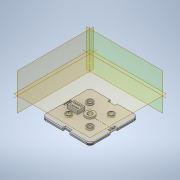
# Autodesk Inventor part: brick_bottom_standard
Saved by Autodesk Inventor 2021 (Build 250183000, 183)
## iProperties
Created: 2025-08-13
Part Number: brick_bottom_standard
Material: Generisch
Document SubType Name: Modeling
Designer: pasca
Density: 1 g/cm^3
Appearance: Vorgabe
Author: pasca
Autodesk Inventor part; units mm, degrees
sketch "Skizze1" plane through (27.583261, -56.113234, -10.899999) normal (0, 0, 1) x (1, 0, 0)
  line L0 (20.486741, 28.426785) -> (20.486741, 31.173234)
  line L1 (28.486738, 28.426785) -> (20.486741, 28.426785)
  line L2 (28.486738, 31.173234) -> (28.486738, 28.426785)
  circle A0 centre (48.116381, 27.672954) radius 3.500451
  line L3 (48.870292, 0.100002) -> (48.870292, 7.94323)
  line L4 (48.973479, 8.043232) -> (51.613555, 8.043232)
  line L5 (51.613555, 0) -> (48.973479, 0)
  circle A1 centre (48.116472, -19.586583) radius 3.50032
  line L6 (20.529933, -20.340319) -> (28.529944, -20.340319)
  line L7 (28.529944, -20.340319) -> (28.529944, -23.086762)
  line L8 (20.529933, -23.086762) -> (20.529933, -20.340319)
  circle A2 centre (0.857019, -19.586408) radius 3.500451
  line L9 (0.103188, 7.94323) -> (0.103188, 0.100002)
  line L10 (-2.640073, 8.043232) -> (0, 8.043232)
  line L11 (0, 0) -> (-2.640073, 0)
  circle A3 centre (0.856903, 27.67302) radius 3.50027
  circle A4 centre (6.691673, 3.973123) radius 1.000129
  circle A5 centre (9.236925, 3.973204) radius 1.000185
  circle A6 centre (11.781701, 3.973221) radius 0.999961
  circle A7 centre (14.326498, 3.973153) radius 0.999748
  circle A8 centre (14.3269, 0.233503) radius 0.99969
  circle A9 centre (11.78165, 0.233145) radius 1.000125
  circle A10 centre (9.236749, 0.233322) radius 0.999912
  circle A11 centre (6.691637, 0.232928) radius 1.000319
  line L12 (-2.640073, 8.043232) -> (0.103188, 8.043232)
  line L13 (0.103188, 8.043232) -> (0.103188, 0)
  line L14 (0.103188, 0) -> (-2.640073, 0)
  line L15 (20.486741, 31.173234) -> (20.486741, 28.426785)
  line L16 (28.486738, 28.426785) -> (28.486738, 31.173234)
  line L17 (48.116736, 31.173234) -> (28.486738, 31.173234)
  line L18 (0.85674, -23.086762) -> (20.529933, -23.086762)
  line L19 (-2.643261, 0.100002) -> (-2.643261, -19.586763)
  line L20 (51.616735, -19.586763) -> (51.616735, 0.100002)
  line L21 (-2.643261, 27.673233) -> (-2.643261, 7.94323)
  line L22 (20.486741, 31.173234) -> (0.85674, 31.173234)
  line L23 (51.616735, 7.94323) -> (51.616735, 27.673233)
  line L24 (28.529944, -23.086762) -> (48.116736, -23.086762)
  line L25 (-2.643261, -23.086762) -> (51.616735, -23.086762)
  line L26 (51.616735, -23.086762) -> (51.616735, 31.173234)
  line L27 (51.616735, 31.173234) -> (-2.643261, 31.173234)
  line L28 (-2.643261, 31.173234) -> (-2.643261, -23.086762)
  line L29 (51.613555, 8.043232) -> (48.870292, 8.043232)
  line L30 (48.870292, 8.043232) -> (48.870292, 0)
  line L31 (48.870292, 0) -> (51.613555, 0)
  line L32 (48.870292, 0) -> (51.613555, 0)
  line L33 (48.870292, 0) -> (48.870292, 8.043232)
  line L34 (51.613555, 8.043232) -> (48.870292, 8.043232)
  line L35 (48.870292, 8.043232) -> (48.870292, 0)
  line L36 (48.870292, 0) -> (51.613555, 0)
  line L37 (51.613555, 0) -> (51.613555, 8.043232)
  line L38 (0.103188, 0) -> (-2.640073, 0)
  line L39 (-2.640073, 8.043232) -> (0.103188, 8.043232)
  line L40 (0.103188, 0) -> (-2.640073, 0)
  line L41 (-2.640073, 0) -> (-2.640073, 8.043232)
  line L42 (-2.640073, 8.043232) -> (0.103188, 8.043232)
  line L43 (0.103188, 8.043232) -> (0.103188, 0)
  point P0 (-27.583261, 56.113234)
  point P1 (0.837182, 31.173234)
  point P2 (-2.643261, 27.700217)
  point P3 (-2.643261, -19.621008)
  point P4 (0.830931, -23.086762)
  point P5 (48.147826, -23.086762)
  point P6 (51.616735, -19.606381)
  point P7 (51.616735, 27.699042)
  point P8 (48.150981, 31.173234)
  constraints: 48 end point, 6 perpendicular, 5 collinear, 4 horizontal, 4 parallel, 3 point on line, 1 vertical
sketch "Skizze1 outline for Extrusion2" plane through (27.583261, -56.113234, -10.899999) normal (0, 0, 1) x (1, 0, 0)
  line L0 (28.486738, 28.426785) -> (20.486741, 28.426785)
  line L1 (28.486738, 31.173234) -> (28.486738, 28.426785)
  line L2 (20.486741, 28.426785) -> (20.486741, 31.173234)
  line L3 (48.116736, 31.173234) -> (28.486738, 31.173234)
  line L4 (20.486741, 31.173234) -> (0.85674, 31.173234)
  line L5 (48.150981, 31.173234) -> (48.116736, 31.173234)
  line L6 (0.85674, 31.173234) -> (0.837182, 31.173234)
  arc A0 (51.616735, 27.699042) -> (48.150981, 31.173234) centre (48.116381, 27.672954) ccw
  arc A1 (0.837182, 31.173234) -> (-2.643261, 27.700217) centre (0.856903, 27.67302) ccw
  line L7 (51.616735, 27.673233) -> (51.616735, 27.699042)
  line L8 (-2.643261, 27.700217) -> (-2.643261, 27.673233)
  line L9 (51.616735, 7.94323) -> (51.616735, 27.673233)
  line L10 (-2.643261, 27.673233) -> (-2.643261, 7.94323)
  line L11 (51.616735, 0.100002) -> (51.616735, 7.94323)
  line L12 (-2.643261, 7.94323) -> (-2.643261, 0.100002)
  line L13 (51.616735, -19.586763) -> (51.616735, 0.100002)
  line L14 (-2.643261, 0.100002) -> (-2.643261, -19.586763)
  line L15 (51.616735, -19.606381) -> (51.616735, -19.586763)
  line L16 (-2.643261, -19.586763) -> (-2.643261, -19.621008)
  arc A2 (48.147826, -23.086762) -> (51.616735, -19.606381) centre (48.116472, -19.586583) ccw
  arc A3 (-2.643261, -19.621008) -> (0.830931, -23.086762) centre (0.857019, -19.586408) ccw
  line L17 (48.116736, -23.086762) -> (48.147826, -23.086762)
  line L18 (0.830931, -23.086762) -> (0.85674, -23.086762)
  line L19 (28.529944, -23.086762) -> (48.116736, -23.086762)
  line L20 (0.85674, -23.086762) -> (20.529933, -23.086762)
  line L21 (28.529944, -20.340319) -> (28.529944, -23.086762)
  line L22 (20.529933, -23.086762) -> (20.529933, -20.340319)
  line L23 (20.529933, -20.340319) -> (28.529944, -20.340319)
  circle A4 centre (6.691637, 0.232928) radius 1.000319
  circle A5 centre (9.236749, 0.233322) radius 0.999912
  circle A6 centre (11.78165, 0.233145) radius 1.000125
  circle A7 centre (14.3269, 0.233503) radius 0.99969
  line L24 (-2.640073, 0) -> (-2.640073, 8.043232)
  line L25 (0, 0) -> (-2.640073, 0)
  line L26 (0.103188, 0) -> (0, 0)
  line L27 (0.103188, 0.100002) -> (0.103188, 0)
  line L28 (0.103188, 7.94323) -> (0.103188, 0.100002)
  line L29 (0.103188, 8.043232) -> (0.103188, 7.94323)
  line L30 (0, 8.043232) -> (0.103188, 8.043232)
  line L31 (-2.640073, 8.043232) -> (0, 8.043232)
  circle A8 centre (6.691673, 3.973123) radius 1.000129
  circle A9 centre (9.236925, 3.973204) radius 1.000185
  circle A10 centre (11.781701, 3.973221) radius 0.999961
  circle A11 centre (14.326498, 3.973153) radius 0.999748
  line L32 (51.613555, 8.043232) -> (51.613555, 0)
  line L33 (48.973479, 8.043232) -> (51.613555, 8.043232)
  line L34 (48.870292, 8.043232) -> (48.973479, 8.043232)
  line L35 (48.870292, 7.94323) -> (48.870292, 8.043232)
  line L36 (48.870292, 0.100002) -> (48.870292, 7.94323)
  line L37 (48.870292, 0) -> (48.870292, 0.100002)
  line L38 (48.973479, 0) -> (48.870292, 0)
  line L39 (51.613555, 0) -> (48.973479, 0)
extrude "Extrusion2" add sketch "Skizze1 outline for Extrusion2" along normal blind 1.8
sketch "Skizze2" plane through (27.583261, -56.113234, -9.099999) normal (0, 0, 1) x (1, 0, 0)
  line L0 (4.491739, -1.966767) -> (16.526742, -1.966767)
  line L1 (4.491739, -1.966767) -> (4.491739, 6.173234)
  line L2 (16.526742, 6.173234) -> (16.526742, -1.966767)
  line L3 (4.491739, 6.173234) -> (16.526742, 6.173234)
  line L4 (16.526742, -1.966767) -> (4.491739, -1.966767)
  circle A0 centre (9.236925, 3.973204) radius 1.000185
  circle A1 centre (11.781802, 3.973293) radius 1.000086
  circle A2 centre (14.32665, 3.9735) radius 1.00028
  circle A3 centre (14.326722, 0.233403) radius 0.999832
  circle A4 centre (11.78165, 0.233145) radius 1.000125
  circle A5 centre (9.236749, 0.233322) radius 0.999912
  circle A6 centre (6.691673, 3.973123) radius 1.000129
  circle A7 centre (6.691637, 0.232928) radius 1.000319
  point P0 (-27.583261, 56.113234)
extrude "Extrusion3" add sketch "Skizze2" along normal blind 4
sketch "Skizze3" plane through (27.583261, -56.113234, -9.099999) normal (0, 0, 1) x (1, 0, 0)
  circle A0 centre (12.321135, -8.122127) radius 2.666057
  circle A1 centre (12.321681, -8.121848) radius 3.499995
  circle A2 centre (12.3219, -8.121781) radius 2.666437
  circle A3 centre (12.321203, -8.121912) radius 3.500477
  circle A4 centre (24.486223, 4.041641) radius 4.998329
  circle A5 centre (24.486657, 4.043031) radius 2.66645
  circle A6 centre (36.651848, 16.208558) radius 2.666928
  circle A7 centre (36.651807, 16.208589) radius 3.500291
  line L0 (51.613555, 8.043232) -> (51.613555, 0)
  line L1 (51.613555, 4.021616) -> (-2.640073, 4.021616) construction
  line L2 (-2.640073, 0) -> (-2.640073, 8.043232)
  circle A8 centre (12.321135, 16.165359) radius 2.666057
  circle A9 centre (12.321203, 16.165144) radius 3.500477
  circle A10 centre (36.651848, -8.165326) radius 2.666928
  circle A11 centre (36.651807, -8.165357) radius 3.500291
  point P0 (-27.583261, 56.113234)
  point P1 (10.243668, -6.451202)
  point P2 (12.201311, -10.78549)
  constraints: 4 centre point, 4 symmetric about line, 2 end point, 2 midpoint, 4 other
extrude "Extrusion4" add sketch "Skizze3" along normal blind 2
sketch "Skizze4" plane through (27.583261, -56.113234, -9.099999) normal (0, 0, 1) x (1, 0, 0)
  line L0 (51.616735, -19.606381) -> (51.616735, 27.699042) construction
  line L1 (51.616735, 4.04633) -> (-2.640073, 4.021616) construction
  line L2 (-2.640073, 0) -> (-2.640073, 8.043232) construction
  circle A0 centre (36.651848, 16.208558) radius 2.666928 construction
  circle A1 centre (36.651807, 16.208589) radius 3.500291 construction
  circle A2 centre (12.321681, -8.121848) radius 3.499995 construction
  arc A3 (12.201311, -10.78549) -> (10.243668, -6.451202) centre (12.3219, -8.121781) ccw construction
  arc A4 (10.243668, -6.451202) -> (12.201311, -10.78549) centre (12.321135, -8.122127) ccw construction
  circle A5 centre (24.486657, 4.043031) radius 2.66645 construction
  circle A6 centre (36.651848, 16.208558) radius 2.666928 construction
  arc A7 (10.243668, -6.451202) -> (12.201311, -10.78549) centre (12.321135, -8.122127) ccw construction
  arc A8 (12.201311, -10.78549) -> (10.243668, -6.451202) centre (12.3219, -8.121781) ccw construction
  point P0 (-27.583261, 56.113234)
  constraints: 2 end point, 2 midpoint
